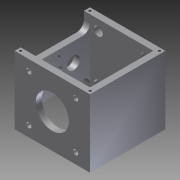
# Autodesk Inventor part: 1_0204_002
Saved by Autodesk Inventor 2012 SP1 (Build 160190100, 190)
## iProperties
Created: 2013-03-22
Part Number: 1_0204_002
Material: Default
Document SubType Name: Modeling
Designer: vogel
Density: 1 g/cm^3
Author: vogel
Autodesk Inventor part; units mm, degrees
note: some values were not read from the file. Chosen so that the rebuilt part matches the saved one: direction of "Bohrung6"; direction of "Bohrung7"; direction of "Bohrung8".
ref_plane "YZ Plane" through (0, 0, 0) normal (1, 0, 0) x (0, 1, 0)
ref_plane "XZ Plane" through (0, 0, 0) normal (0, 1, 0) x (-1, 0, 0)
sketch "Skizze1" plane through (0, 0, 0) normal (0, 0, 1) x (1, 0, 0)
  line L0 (-25, 25) -> (25, 25)
  line L1 (25, 25) -> (25, -25)
  line L2 (25, -25) -> (-25, -25)
  line L3 (-25, -25) -> (-25, 25)
  line L4 (-35, 0) -> (35, 0) projected
  line L5 (0, -35) -> (0, 35) projected
  line L6 (21, 21) -> (-21, 21)
  line L7 (-21, 21) -> (-21, -21)
  line L8 (-21, -21) -> (21, -21)
  line L9 (21, -21) -> (21, 21)
  point P0 (0, 0)
  dimension "d0" = 50
  dimension "d1" = 50
  dimension "d2" = 4
  constraints: 16 end point, 4 parallel, 2 perpendicular, 1 horizontal, 5 other
  measures "d0" distance between parallel lines of L2 L0
  measures "d1" distance between parallel lines of L1 L3
  measures "d2" distance between parallel lines of L0 L6
extrude "Extrusion1" add sketch "Skizze1" along normal blind 45 contours L0 L5 L6 L7 L4 L3 | L0 L1 L4 L9 L6 L5 | L4 L7 L8 L5 L2 L3 | L1 L2 L5 L8 L9 L4
sketch "Skizze2" plane through (-25, -25, 0) normal (-1, 0, 0) x (0, 0, 1)
  line L0 (0, 50) -> (45, 50) projected
  line L1 (0, 0) -> (45, 0) projected
  line L2 (22.5, 50) -> (22.5, 0)
  line L3 (0, 46) -> (45, 46) projected
  line L4 (0, 4) -> (45, 4) projected
  line L5 (0, 46) -> (5, 46)
  line L6 (10, 41) -> (10, 9)
  line L7 (5, 4) -> (0, 4)
  line L8 (0, 4) -> (0, 46)
  line L9 (45, 4) -> (40, 4)
  line L10 (35, 9) -> (35, 41)
  line L11 (40, 46) -> (45, 46)
  line L12 (45, 46) -> (45, 4)
  arc A0 (40, 46) -> (35, 41) centre (40, 41) ccw
  arc A1 (35, 9) -> (40, 4) centre (40, 9) ccw
  arc A2 (5, 4) -> (10, 9) centre (5, 9) ccw
  arc A3 (10, 41) -> (5, 46) centre (5, 41) ccw
  point P0 (0, 25)
  point P1 (10, 4)
  point P2 (35, 46)
  dimension "d5" = 25
  dimension "d6" = 5
  constraints: 18 end point, 8 point on circle, 8 tangent, 6 point on line, 4 centre point, 4 parallel, 3 equal radius, 2 horizontal, 2 midpoint, 2 perpendicular, 1 other
  measures "d5" distance between parallel lines of L6 L10
  measures "d6" radius of A0
extrude "Extrusion2" cut sketch "Skizze2" against normal up to surface (46 mm away) contours A3 L6 A2 L4 L8 L3 | L3 L12 L4 A1 L10 A0
sketch "Skizze4" plane through (-25, -25, 0) normal (0, -1, 0) x (1, 0, 0)
  line L0 (50, 45) -> (0, 45) projected
  line L1 (0, 0) -> (0, 45) projected
  line L2 (50, 0) -> (50, 45) projected
  line L3 (0, 22.5) -> (50, 22.5)
  line L4 (25, 45) -> (25, 0)
  circle A0 centre (25, 22.5) radius 11
  dimension "d19" = 22
  constraints: 4 end point, 4 midpoint, 1 centre point, 1 perpendicular
  measures "d19" diameter of A0
extrude "Extrusion3" cut sketch "Skizze4" against normal up to surface (46 mm away) contours A0 L3 L4 | L4 L3 A0 | A0 L4 L3 | L4 A0 L3
mirror "Spiegeln1" about plane through (0, 0, 0) normal (0, 0, 1) of "Extrusion1", "Extrusion2", "Extrusion3"
sketch "Skizze5" plane through (-25, 25, 45) normal (0, 1, 0) x (1, 0, 0)
  circle A0 centre (33.6603, 27.5) radius 3.45 projected
  circle A1 centre (16.3397, 27.5) radius 3.45 projected
  circle A2 centre (25, 12.5) radius 3.45 projected
  line L0 (0, 0) -> (50, 0) projected
  line L1 (50, 0) -> (50, 90) projected
  line L2 (60, 45) -> (-10, 45) projected
  line L3 (50, 45) -> (0, 45)
  line L4 (0, 45) -> (0, 0)
  line L5 (0, 0) -> (50, 0)
  line L6 (50, 0) -> (50, 45)
  point P0 (25, 45)
  constraints: 8 end point, 2 parallel, 1 horizontal, 1 midpoint, 1 perpendicular, 1 point on line
extrude "Extrusion4" cut sketch "Skizze5" against normal through all contours A0 | A1 | A2 | L4 L2 L1 L0
sketch "Skizze10" plane through (-25, -16, -10) normal (-1, 0, 0) x (0, 0, 1)
  circle A0 centre (-20.5, 16) radius 1.7 projected
  circle A1 centre (-4.5, 16) radius 1.7 projected
  point P0 (10, 16)
  constraints: 2 coincident
hole "Bohrung6" at (-25, 0, -14.5) at (-25, 0, -30.5) direction (1, 0, 0) diameter 2.459 end up to surface thread size "M3x0.5" class "6H" standard "ISO Metric profile"
sketch "Skizze11" plane through (-25, -16, -10) normal (-1, 0, 0) x (0, 0, 1)
  line L0 (0, 0) -> (0, 32) projected
  line L1 (-35, 41) -> (10, 41) projected
  line L2 (-25, 32) -> (-25, 0) projected
  line L3 (10, -9) -> (-35, -9) projected
  line L4 (-12.5, 41) -> (-12.5, -9)
  line L5 (0, 16) -> (-25, 16)
  point P0 (10, 16)
  point P1 (-12.5, 16)
  constraints: 5 midpoint, 4 end point
hole "Bohrung7" at (-25, 0, -22.5) direction (1, 0, 0) diameter 5.5 end up to surface
sketch "Skizze12" plane through (-25, -16, -10) normal (-1, 0, 0) x (0, 0, 1)
  line L0 (0, 0) -> (0, 32) projected
  line L1 (-35, 41) -> (10, 41) projected
  line L2 (-25, 32) -> (-25, 0) projected
  line L3 (10, -9) -> (-35, -9) projected
  line L4 (-12.5, 41) -> (-12.5, -9)
  line L5 (-25, 16) -> (0, 16)
  point P0 (10, 16)
  point P1 (-12.5, 26)
  point P2 (-12.5, 6)
  dimension "d67" = 20
  constraints: 4 end point, 4 midpoint, 2 point on line, 1 symmetric about line
  measures "d67" distance of point (-12.5, 6) point (-12.5, 26)
hole "Bohrung8" at (-25, 10, -22.5) at (-25, -10, -22.5) direction (1, 0, 0) diameter 8.5 end up to surface
sketch "Skizze13" plane through (-25, -25, -45) normal (0, -1, 0) x (1, 0, 0)
  circle A0 centre (25, 22.5) radius 11 projected
  line L0 (-10, 45) -> (60, 45) projected
  line L1 (25, 54) -> (25, -9) projected
  line L2 (9.5, 38) -> (40.5, 38)
  line L3 (40.5, 38) -> (40.5, 7)
  line L4 (40.5, 7) -> (9.5, 7)
  line L5 (9.5, 7) -> (9.5, 38)
  line L6 (25, 22.5) -> (30.7516, 22.5)
  point P0 (25, 45)
  dimension "d75" = 31
  constraints: 10 end point, 4 coincident, 3 perpendicular, 2 parallel, 1 horizontal, 2 other
  measures "d75" distance of L2.start L2.end
hole "Bohrung9" at (-15.5, -25, -7) at (15.5, -25, -7) at (15.5, -25, -38) at (-15.5, -25, -38) direction (0, 1, 0) diameter 3.4 end through all
sketch "Skizze14" plane through (-25, 25, -45) normal (0, 1, 0) x (1, 0, 0)
  circle A0 centre (9.5, -7) radius 1.7 projected
  circle A1 centre (40.5, -7) radius 1.7 projected
  circle A2 centre (40.5, -38) radius 1.7 projected
  circle A3 centre (9.5, -38) radius 1.7 projected
  point P0 (25, -45)
  constraints: 4 coincident
hole "Bohrung10" at (-15.5, 25, -38) at (15.5, 25, -38) at (15.5, 25, -7) at (-15.5, 25, -7) direction (0, -1, 0) diameter 6 depth 8 tip angle 118
sketch "Skizze15" plane through (-25, 25, 0) normal (0, 0, 1) x (1, 0, 0)
  line L0 (0, -50) -> (0, -46) projected
  line L1 (50, -50) -> (0, -50) projected
  line L2 (50, 0) -> (50, -50) projected
  line L3 (0, 0) -> (50, 0) projected
  line L4 (2, -2) -> (48, -2)
  line L5 (48, -2) -> (48, -48)
  line L6 (48, -48) -> (2, -48)
  line L7 (2, -48) -> (2, -2)
  point P0 (25, -25)
  dimension "d90" = 2
  dimension "d91" = 2
  dimension "d92" = 2
  dimension "d93" = 2
  constraints: 8 end point, 4 coincident, 2 parallel, 1 horizontal, 1 perpendicular
  measures "d90" distance between parallel lines of L4 L3
  measures "d91" distance between parallel lines of L2 L5
  measures "d92" distance between parallel lines of L6 L1
  measures "d93" distance between parallel lines of L0 L7
hole "Bohrung11" at (-23, 23, 0) at (23, 23, 0) at (23, -23, 0) at (-23, -23, 0) direction (0, 0, -1) diameter 1.567 depth 8 tip angle 118 thread size "M2x0.4" class "6H" standard "ISO Metric profile"
ref_plane "Arbeitsebene1" through (-25, 25, -22.5) normal (0, 0, 1) x (1, 0, 0)
mirror "Spiegeln2" about plane through (-25, 25, -22.5) normal (0, 0, 1) of "Bohrung11"
